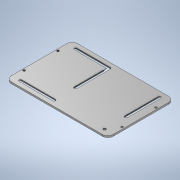
# Autodesk Inventor part: PlateAxial
Saved by Autodesk Inventor 2022 (Build 260153000, 153)
## iProperties
Created: 2022-12-14
Part Number: PlateAxial
Material: Aluminum, Anodized Silver
Document SubType Name: Modeling
Designer: braxt
Density: 2.7 g/cm^3
Appearance: Anodized - Light Gray
Author: braxt
Autodesk Inventor part; units mm, degrees
ref_plane "YZ Plane" through (0, 0, 0) normal (1, 0, 0) x (0, 1, 0)
ref_plane "XZ Plane" through (0, 0, 0) normal (0, 1, 0) x (-1, 0, 0)
sketch "Sketch1" plane through (0, 0, 0) normal (0, 1, 0) x (-1, 0, 0)
  line L0 (-301.6, 175.65) -> (-203.3004, 175.65)
  line L1 (-203.3004, 275.65) -> (-301.6, 275.65)
  line L2 (-301.6, 275.65) -> (-301.6, 175.65)
  line L3 (-301.6, 275.65) -> (-201.6, 275.65)
  line L4 (-201.6, 275.65) -> (-201.6, 175.65)
  line L5 (-201.6, 175.65) -> (-301.6, 175.65)
  line L6 (-301.6, 175.65) -> (-301.6, 275.65)
  line L7 (-301.6, 175.65) -> (-301.6, 275.65)
  line L8 (-301.6, 275.65) -> (-201.6, 275.65)
  line L9 (-201.6, 275.65) -> (-201.6, 75.65)
  line L10 (-301.6, 75.65) -> (-301.6, 275.65)
  line L11 (-301.6, 75.65) -> (-301.6, 275.65)
  line L12 (-152.1, 75.65) -> (-162.1, 75.65)
  line L13 (-157.1, 260.65) -> (-57.1, 260.65)
  line L14 (-52.1, 265.65) -> (-52.1, 265.65)
  line L15 (-57.1, 270.65) -> (-157.1, 270.65)
  circle A0 centre (-346.1, 265.65) radius 5
  arc A1 (-157.1, 270.65) -> (-157.1, 260.65) centre (-157.1, 265.65) ccw
  line L16 (-201.6, 75.65) -> (-157.1, 75.65)
  arc A2 (-152.1, 185.65) -> (-162.1, 185.65) centre (-157.1, 185.65) ccw
  line L17 (-162.1, 185.65) -> (-162.1, 85.65)
  line L18 (-152.1, 75.65) -> (-152.1, 185.65)
  line L19 (-157.1, 80.65) -> (-157.1, 80.65)
  arc A3 (-341.1, 185.65) -> (-351.1, 185.65) centre (-346.1, 185.65) ccw
  line L20 (-341.1, 85.65) -> (-341.1, 185.65)
  line L21 (-351.1, 185.65) -> (-351.1, 85.65)
  line L22 (-346.1, 80.65) -> (-346.1, 80.65)
  line L23 (-301.6, 275.65) -> (-201.6, 275.65)
  line L24 (-201.6, 275.65) -> (-201.6, 49.35)
  line L25 (-201.6, 49.35) -> (-301.6, 49.35)
  line L26 (-301.6, 49.35) -> (-301.6, 275.65)
  line L27 (-351.1, 85.65) -> (-351.1, 59.35)
  line L28 (-341.1, 59.35) -> (-341.1, 85.65)
  arc A4 (-351.1, 59.35) -> (-341.1, 59.35) centre (-346.1, 59.35) ccw
  line L29 (-152.1, 80.65) -> (-152.1, 64.35)
  line L30 (-162.1, 59.35) -> (-162.1, 85.65)
  arc A5 (-162.1, 59.35) -> (-157.1, 54.35) centre (-157.1, 59.35) ccw
  line L31 (-301.6, 49.35) -> (-75.3, 49.35)
  line L32 (-75.3, 49.35) -> (-75.3, 275.65)
  line L33 (-75.3, 275.65) -> (-201.6, 275.65)
  line L34 (-157.1, 54.35) -> (-30.8, 54.35)
  arc A6 (-30.8, 54.35) -> (-30.8, 64.35) centre (-30.8, 59.35) ccw
  line L35 (-30.8, 64.35) -> (-152.1, 64.35)
  line L36 (-57.1, 260.65) -> (-30.8, 260.65)
  line L37 (-57.1, 270.65) -> (-30.8, 270.65)
  arc A7 (-30.8, 260.65) -> (-30.8, 270.65) centre (-30.8, 265.65) ccw
  line L38 (-69.2464, 270.65) -> (-69.2464, 286.45)
  line L39 (2.2, 286.45) -> (-379.1, 286.45)
  line L40 (-52.1, 54.35) -> (-52.1, 38.55)
  line L41 (2.2, 38.55) -> (-379.1, 38.55)
  line L42 (-25.8, 59.35) -> (-4.8, 59.35)
  line L43 (2.2, 38.55) -> (2.2, 286.45)
  line L44 (-4.8, 99) -> (-4.8, 226)
  line L45 (-372.1, 99) -> (-372.1, 226)
  line L46 (-379.1, 38.55) -> (-379.1, 286.45)
  point P0 (-52.1, 270.65)
  point P1 (-52.1, 260.65)
  point P2 (-157.1, 85.65)
  point P3 (-157.1, 185.65)
  point P4 (-157.1, 85.65)
  point P5 (-162.1, 80.65)
  point P6 (0, 305)
  point P7 (-152.1, 75.65)
  dimension "d2" = 100
  dimension "d3" = 100
  dimension "d7" = 10
  dimension "d8" = 10
  dimension "d16" = 10
  dimension "d17" = 44.5
  dimension "d20" = 10
  dimension "d21" = 10
  dimension "d22" = 10
  dimension "d70" = 226.3
  dimension "d72" = 10
  dimension "d73" = 10
  dimension "d180" = 226.3
  dimension "d224" = 15.8
  dimension "d227" = 15.8
  dimension "d229" = 21
  dimension "d233" = 127
  dimension "d235" = 127
  constraints: 94 end point, 15 point on circle, 12 parallel, 10 horizontal, 10 perpendicular, 10 point on line, 8 centre point, 2 vertical, 1 midpoint, 1 tangent
  measures "d2" distance of L5.start L5.end
  measures "d3" distance of L3.end L5.start
  measures "d7" distance of point (-52.1, 270.65) point (-52.1, 260.65)
  measures "d8" diameter of A0
  measures "d16" diameter of A1
  measures "d17" distance of L9.end L16.end
  measures "d20" distance of L29.start point (-162.1, 80.65)
  measures "d21" diameter of A2
  measures "d22" diameter of A3
  measures "d70" distance of L23.end L24.end
  measures "d72" diameter of A4
  measures "d73" diameter of A5
  measures "d180" distance of L25.end L31.end
  measures "d224" distance of L38.start L38.end
  measures "d227" distance of L40.start L40.end
  measures "d229" distance of L42.start L42.end
  measures "d233" distance of L44.start L44.end
  measures "d235" distance of L45.start L45.end
extrude "Extrusion1" add sketch "Sketch1" along normal blind 3.175 contours L2 L1 L3 L4 L5 L0 | L10 L26 L25 L31 L32 L34 L40 L41 L46 L39 L38 L15 L33 L3 L1 L2 | L0 L5 L9 L24 L25 L26 L10 | L4 L33 L32 L15 A1 L13 L35 L29 L18 A2 L17 L30 L16 L9 | L16 L30 A5 L34 L32 L31 L24 | L38 L39 L43 L41 L40 L34 A6 L35 L32 L13 L36 A7 L37 L15
sketch "Sketch2" plane through (0, 0, 0) normal (0, -1, 0) x (1, 0, 0)
  line L0 (346.1, 80.65) -> (346.1, 80.65)
  line L1 (353.1, 85.65) -> (353.1, 190.65)
  line L2 (339.1, 190.65) -> (339.1, 85.65)
  line L3 (339.1, 85.65) -> (339.1, 54.35)
  line L4 (353.1, 54.35) -> (353.1, 85.65)
  circle A0 centre (346.1, 265.65) radius 7.25
  line L5 (57.1, 258.65) -> (162.1, 258.65)
  line L6 (162.1, 272.65) -> (57.1, 272.65)
  line L7 (57.1, 272.65) -> (25.8, 272.65)
  line L8 (25.8, 258.65) -> (57.1, 258.65)
  line L9 (25.8, 59.35) -> (25.8, 59.35)
  line L10 (157.1, 190.65) -> (157.1, 190.65)
  line L11 (152.1, 185.65) -> (152.1, 64.35) projected
  line L12 (25.8, 52.35) -> (157.1, 52.35)
  arc A1 (157.1, 52.35) -> (164.1, 59.35) centre (157.1, 59.35) ccw
  line L13 (164.1, 59.35) -> (164.1, 190.65)
  line L14 (150.1, 190.65) -> (150.1, 73.35)
  line L15 (143.1, 66.35) -> (25.8, 66.35)
  arc A2 (143.1, 66.35) -> (150.1, 73.35) centre (143.1, 73.35) ccw
  line L16 (346.1, 185.65) -> (346.1, 190.65)
  arc A3 (353.1, 190.65) -> (339.1, 190.65) centre (346.1, 190.65) ccw
  arc A4 (339.1, 54.35) -> (353.1, 54.35) centre (346.1, 54.35) ccw
  arc A5 (164.1, 190.65) -> (150.1, 190.65) centre (157.1, 190.65) ccw
  arc A6 (25.8, 66.35) -> (25.8, 52.35) centre (25.8, 59.35) ccw
  arc A7 (30.8, 270.65) -> (30.8, 260.65) centre (30.8, 265.65) ccw projected
  arc A8 (25.8, 272.65) -> (25.8, 258.65) centre (25.8, 265.65) ccw
  arc A9 (162.1, 258.65) -> (162.1, 272.65) centre (162.1, 265.65) ccw
  point P0 (0, 305)
  point P1 (52.1, 260.65)
  dimension "d209" = 7
  dimension "d212" = 5
  dimension "d213" = 14
  dimension "d215" = 14
  dimension "d217" = 14
  dimension "d219" = 14
  dimension "d221" = 14
  dimension "d223" = 14
  constraints: 32 end point, 16 point on circle, 9 centre point, 3 coincident, 2 tangent, 1 horizontal, 1 vertical
  measures "d209" radius of A2
  measures "d212" distance of L16.start L16.end
  measures "d213" diameter of A3
  measures "d215" diameter of A4
  measures "d217" diameter of A5
  measures "d219" diameter of A6
  measures "d221" diameter of A8
  measures "d223" diameter of A9
extrude "Extrusion2" cut sketch "Sketch2" against normal blind 2
sketch "Sketch4" plane through (0, 0, 0) normal (0, -1, 0) x (1, 0, 0)
  line L0 (339.1, 54.35) -> (339.1, 190.65) projected
  line L1 (353.1, 190.65) -> (353.1, 54.35) projected
  line L2 (150.1, 73.35) -> (150.1, 190.65) projected
  line L3 (164.1, 190.65) -> (164.1, 59.35) projected
  arc A0 (157.1, 52.35) -> (164.1, 59.35) centre (157.1, 59.35) ccw projected
  line L4 (157.1, 52.35) -> (25.8, 52.35) projected
  arc A1 (143.1, 66.35) -> (150.1, 73.35) centre (143.1, 73.35) ccw projected
  line L5 (25.8, 66.35) -> (143.1, 66.35) projected
  circle A2 centre (346.1, 265.65) radius 7.25 projected
  line L6 (162.1, 258.65) -> (25.8, 258.65) projected
  line L7 (25.8, 272.65) -> (162.1, 272.65) projected
  arc A3 (339.1, 54.35) -> (353.1, 54.35) centre (346.1, 54.35) ccw projected
  arc A4 (353.1, 190.65) -> (339.1, 190.65) centre (346.1, 190.65) ccw projected
  arc A5 (164.1, 190.65) -> (150.1, 190.65) centre (157.1, 190.65) ccw projected
  arc A6 (25.8, 66.35) -> (25.8, 52.35) centre (25.8, 59.35) ccw projected
  arc A7 (162.1, 258.65) -> (162.1, 272.65) centre (162.1, 265.65) ccw projected
  arc A8 (25.8, 272.65) -> (25.8, 258.65) centre (25.8, 265.65) ccw projected
  line L8 (-2.2, 286.45) -> (379.1, 286.45) projected
  line L9 (379.1, 38.55) -> (-2.2, 38.55) projected
  line L10 (-2.2, 38.55) -> (-2.2, 286.45) projected
  line L11 (379.1, 286.45) -> (379.1, 38.55) projected
  point P0 (353.1, 59.35)
  point P1 (339.1, 59.35)
  point P2 (339.1, 185.65)
  point P3 (353.1, 185.65)
  point P4 (150.1, 185.65)
  point P5 (164.1, 185.65)
  point P6 (30.8, 52.35)
  point P7 (30.8, 66.35)
  point P8 (157.1, 258.65)
  point P9 (30.8, 258.65)
  point P10 (157.1, 272.65)
  point P11 (30.8, 272.65)
extrude "Extrusion4" add sketch "Sketch4" along normal blind 3.175
fillet "Fillet2" radius 20 4 edges at (-2.2, 0, 286.45) (379.1, 0, 286.45) (379.1, 0, 38.55) (-2.2, 0, 38.55)
ref_plane "Work Plane2" through (0, -3.175, 0) normal (0, -1, 0) x (1, 0, 0)
sketch "Sketch6" plane through (0, -3.175, 0) normal (0, -1, 0) x (1, 0, 0)
  line L0 (4.8, 99) -> (4.8, 226) projected
  line L1 (372.1, 99) -> (372.1, 226) projected
  point P0 (0, 0)
hole "Hole1" at (4.8, -3.175, 226) at (4.8, -3.175, 99) at (372.1, -3.175, 226) at (372.1, -3.175, 99) direction (0, 1, 0) diameter 8 end through all counterbore diameter 12 counterbore depth 5.175
body "Solid1"
